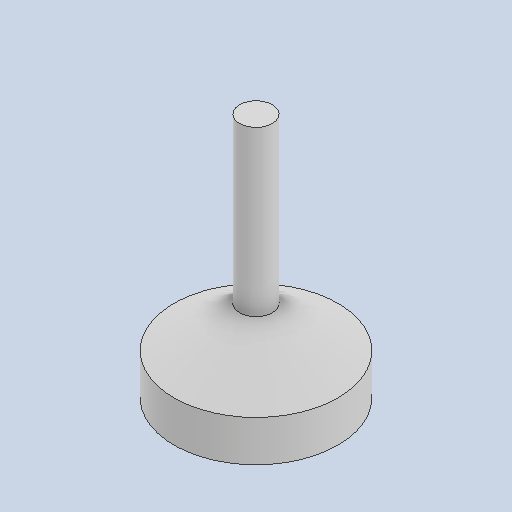
# Autodesk Inventor part: Foot
Saved by Autodesk Inventor 2023 (Build 270158030, 158C)
## iProperties
Created: 2022-07-14
Part Number: Foot
Material: Generic
Document SubType Name: Modeling
Designer: jeremyy
Density: 1 g/cm^3
Appearance: Default
Author: jeremyy
Autodesk Inventor part; units mm, degrees
ref_plane "YZ Plane" through (0, 0, 0) normal (1, 0, 0) x (0, 1, 0)
ref_plane "XZ Plane" through (0, 0, 0) normal (0, 1, 0) x (-1, 0, 0)
ref_plane "XY Plane" through (0, 0, 0) normal (0, 0, 1) x (1, 0, 0)
sketch "Sketch1" plane through (0, 0, 0) normal (0, 0, 1) x (1, 0, 0)
  line L0 (0, 0) -> (12.7, 0)
  line L1 (12.7, 0) -> (12.7, 6.35)
  line L2 (12.7, 6.35) -> (2.54, 12.7)
  line L3 (2.54, 12.7) -> (0, 12.7)
  line L4 (0, 12.7) -> (0, 0)
  line L5 (2.54, 12.7) -> (2.54, 38.1)
  line L6 (2.54, 38.1) -> (0, 38.1)
  line L7 (0, 38.1) -> (0, 0)
  point P0 (0, 12.7)
  dimension "d0" = 12.7
  dimension "d1" = 6.35
  dimension "d2" = 6.35
  dimension "d3" = 2.54
  dimension "d4" = 25.4
  constraints: 16 end point, 4 perpendicular, 1 horizontal, 1 parallel, 1 vertical
  measures "d0" distance of L0.start L0.end
  measures "d1" distance of L0.end L1.end
  measures "d2" vertical distance of L1.end L2.end
  measures "d3" distance of L2.end L3.end
  measures "d4" distance of L2.end L5.end
revolve "Revolution1" add sketch "Sketch1" angle 360 about axis through (0, 38.1, 0) along (0, -1, 0)
body "Solid1"
